# Autodesk Inventor part: 25AA1024_DIP8
Saved by Autodesk Inventor 2015 SP1 (Build 190203100, 203)
## iProperties
Created: 2015-06-25
Part Number: 25AA1024_DIP8
Material: Generic
Document SubType Name: Modeling
Designer: Patrick
Density: 1 g/cm^3
Appearance: DIP760_8, 25AA1024_DIP8
Author: Patrick
Autodesk Inventor part; units mm, degrees
ref_plane "YZ Plane" through (0, 0, 0) normal (1, 0, 0) x (0, 1, 0)
ref_plane "XZ Plane" through (0, 0, 0) normal (0, 1, 0) x (-1, 0, 0)
ref_plane "XY Plane" through (0, 0, 0) normal (0, 0, 1) x (1, 0, 0)
sketch "DIP760_8, 25AA1024_DIP8_255" plane through (0, 0, 0) normal (0, 0, 1) x (1, 0, 0)
  line L0 (-4.55, -5.325) -> (-4.55, 5.325)
  line L1 (-4.55, 5.325) -> (4.55, 5.325)
  line L2 (4.55, 5.325) -> (4.55, -5.325)
  line L3 (4.55, -5.325) -> (-4.55, -5.325)
  constraints: 8 end point
extrude "Extrusion1" add sketch "DIP760_8, 25AA1024_DIP8_255" along normal blind 1
body "Solid1"
